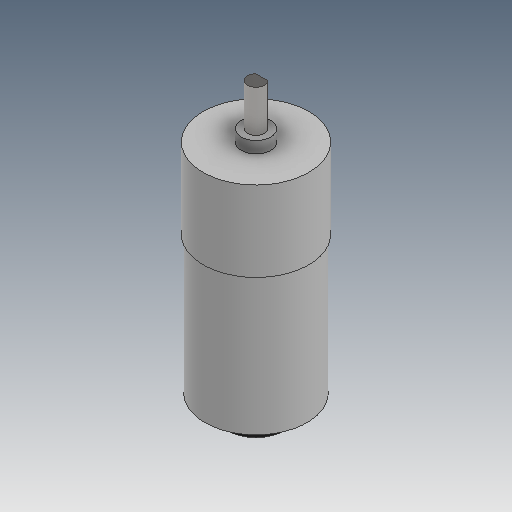
# Autodesk Inventor part: Motor
Saved by Autodesk Inventor 2026.1 (Build 301233020, 233B)
## iProperties
Created: 2025-11-09
Part Number: Motor
Material: Genérico
Document SubType Name: Modeling
Designer: Emmanuel Ribeiro
Density: 1 g/cm^3
Appearance: Padrão
Author: Emmanuel Ribeiro
Autodesk Inventor part; units mm, degrees
ref_plane "YZ Plane" through (0, 0, 0) normal (1, 0, 0) x (0, 1, 0)
ref_plane "XZ Plane" through (0, 0, 0) normal (0, 1, 0) x (-1, 0, 0)
ref_plane "XY Plane" through (0, 0, 0) normal (0, 0, 1) x (1, 0, 0)
sketch "Esboço1" plane through (0, 0, 0) normal (1, 0, 0) x (0, 1, 0)
  line L0 (0, 0) -> (51.1, 0)
  line L1 (51.1, -3.45) -> (51.1, -12.4)
  line L2 (51.1, -12.4) -> (32.3, -12.4)
  line L3 (32.3, -12) -> (0, -12)
  line L4 (32.3, -12.4) -> (32.3, -12)
  line L5 (0, -6.7) -> (-4.3, -6.7)
  line L6 (0, -6.7) -> (0, -12)
  line L7 (-4.3, 0) -> (-4.3, -6.7)
  line L8 (51.1, 0) -> (53.8, 0)
  line L9 (53.8, 0) -> (53.8, -3.45)
  line L10 (53.8, -3.45) -> (51.1, -3.45)
  line L11 (0, 0) -> (-4.3, 0)
  dimension "d0" = 51.1
  dimension "d1" = 12.4
  dimension "d2" = 18.8
  dimension "d4" = 12
  dimension "d5" = 6.7
  dimension "d6" = 4.3
  dimension "d10" = 2.7
  constraints: 24 end point, 4 perpendicular, 3 horizontal, 3 vertical, 1 parallel, 1 point on line
  measures "d0" distance of L0.start L0.end
  measures "d1" distance of L0.end L1.end
  measures "d2" distance of L1.end L2.end
  measures "d4" distance between parallel lines of L0 L3
  measures "d5" distance of L0.start L5.start
  measures "d6" distance of L5.start L5.end
  measures "d10" distance of L8.end L0.end
revolve "Revolução1" add sketch "Esboço1" angle 360 about axis through (0, 0, 0) along (0, 1, 0)
sketch "Esboço2" plane through (0, -4.3, 0) normal (0, -1, 0) x (1, 0, 0)
  circle A0 centre (0, 0) radius 0.95
  dimension "d15" = 1.9
  constraints: 1 centre point, 1 coincident
  measures "d15" diameter of A0
extrude "Extrusão1" add sketch "Esboço2" along normal blind 3.5 separate body
sketch "Esboço3" plane through (0, 53.8, 0) normal (0, 1, 0) x (1, 0, 0)
  circle A0 centre (0, 0) radius 0.95 projected
  arc A1 (-1.4071, 1.35) -> (1.4071, 1.35) centre (0, 0) ccw
  line L0 (-1.4071, 1.35) -> (1.4071, 1.35)
  line L1 (0, 0.95) -> (0, 1.35)
  dimension "d18" = 3.9
  constraints: 4 end point, 2 point on circle, 1 centre point, 1 coincident, 1 horizontal, 1 midpoint, 1 vertical, 1 vertical alignment, 1 other
  measures "d18" diameter of A1
extrude "Extrusão2" add sketch "Esboço3" along normal blind 9.8 separate body contours A0 | L0 A1
